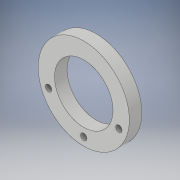
# Autodesk Inventor part: 半円 穴あり
Saved by Autodesk Inventor 2019 (Build 230136000, 136)
## iProperties
Created: 2020-09-25
Part Number: 半円 穴あり
Material: 一般
Document SubType Name: Modeling
Designer: Toshihito
Density: 1 g/cm^3
Appearance: 既定
Mass: 23.499 g
Surface Area: 91.043 cm^2
Volume: 23.499 cm^3
Author: Toshihito
Autodesk Inventor part; units mm, degrees
ref_plane "YZ Plane" through (0, 0, 0) normal (1, 0, 0) x (0, 1, 0)
ref_plane "XZ Plane" through (0, 0, 0) normal (0, 1, 0) x (-1, 0, 0)
ref_plane "XY Plane" through (0, 0, 0) normal (0, 0, 1) x (1, 0, 0)
sketch "スケッチ1" plane through (0, 0, 0) normal (0, 0, 1) x (1, 0, 0)
  arc A0 (-23.45, 0) -> (23.45, 0) centre (0, 0) ccw
  arc A1 (-36.55, 0) -> (36.55, 0) centre (0, 0) ccw
  circle A2 centre (0, -30) radius 2.55
  circle A3 centre (28.1908, -10.2606) radius 2.55
  circle A4 centre (-28.1908, -10.2606) radius 2.55
  line L0 (0, 0) -> (-28.1908, -10.2606) construction
  line L1 (0, 0) -> (28.1908, -10.2606) construction
  line L2 (-48.309, 0) -> (65.7551, 0)
  dimension "d0" = 46.9
  dimension "d1" = 73.1
  dimension "d2" = 5.1
  dimension "d3" = 5.1
  dimension "d4" = 5.1
  dimension "d5" = 30
  dimension "d6" = 30
  dimension "d7" = 30
  dimension "d9" = 20
  dimension "d10" = 20
  constraints: 6 end point, 5 centre point, 4 point on circle, 4 point on line, 3 coincident, 1 horizontal
  measures "d0" diameter of A0
  measures "d1" diameter of A1
  measures "d2" diameter of A2
  measures "d3" diameter of A3
  measures "d4" diameter of A4
  measures "d5" distance of A2.centre point (0, 0)
  measures "d6" distance of L0.start L0.end
  measures "d7" distance of L0.start L1.end
  measures "d9" angle of L2 L0
  measures "d10" angle of L2 L1
extrude "押し出し1" add sketch "スケッチ1" along normal blind 10 contours A0 L2 A1
fillet "フィレット1" radius 2 4 edges at (36.55, 0, 5) (23.45, 0, 5) (-23.45, 0, 5) (-36.55, 0, 5)
sketch "スケッチ3" plane through (0, 0, 10) normal (0, 0, 1) x (1, 0, 0)
  circle A0 centre (0, 0) radius 23.45
  circle A1 centre (0, 0) radius 36.55
  circle A2 centre (28.1908, -10.2606) radius 2.55 projected
  circle A3 centre (28.1908, -10.2606) radius 2.55
  circle A4 centre (0, -30) radius 2.55 projected
  circle A5 centre (0, -30) radius 2.55
  circle A6 centre (-28.1908, -10.2606) radius 2.55 projected
  circle A7 centre (-28.1908, -10.2606) radius 2.55
  constraints: 5 centre point, 5 coincident
extrude "押し出し3" add sketch "スケッチ3" against normal blind 10
